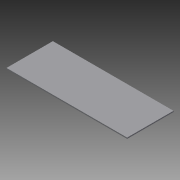
# Autodesk Inventor part: HostPCB
Saved by Autodesk Inventor 2016 (Build 200138000, 138)
## iProperties
Created: 2015-06-09
Part Number: HostPCB
Material: GFRC
Document SubType Name: Modeling
Designer: Yann
Density: 1.7 g/cm^3
Appearance: Flat - Polished Gray
Author: Yann
Autodesk Inventor part; units mm, degrees
ref_plane "YZ Plane" through (0, 0, 0) normal (1, 0, 0) x (0, 1, 0)
ref_plane "XZ Plane" through (0, 0, 0) normal (0, 1, 0) x (-1, 0, 0)
ref_plane "XY Plane" through (0, 0, 0) normal (0, 0, 1) x (1, 0, 0)
sketch "Sketch1" plane through (0, 0, 0) normal (0, 0, 1) x (1, 0, 0)
  line L0 (0, 35) -> (0, -35) construction
  line L1 (-91, 0) -> (91, 0) construction
  line L2 (-65, -25) -> (65, -25)
  line L3 (65, -25) -> (65, 25)
  line L4 (65, 25) -> (-65, 25)
  line L5 (-65, 25) -> (-65, -25)
  line L6 (-65, -25) -> (65, 25) construction
  line L7 (65, -25) -> (-65, 25) construction
  point P0 (0, 0)
  dimension "d0" = 130
  dimension "d1" = 50
  constraints: 12 end point, 2 midpoint, 2 parallel, 1 horizontal, 1 perpendicular
  measures "d0" distance of L4.end L3.end
  measures "d1" distance between parallel lines of L2 L4
extrude "Extrusion1" add sketch "Sketch1" along normal blind 1.2
equation "\"d0\" = HostPCB_Length"
equation "\"d1\" = HostPCB_Width"
equation "\"d2\" = HostPCB_Thickness"
equation "\"Heatsink_Thickness\" = 5"
equation "\"Heatsink_Width\" = 65"
equation "\"Cover_Thickness\" = 2"
equation "\"PowerPCB_Minus_Height\" = 1.2"
equation "\"PowerPCB_Width\" = 63"
equation "\"Interface_Thickness\" = 7"
equation "\"PowerPCB_Thickness\" = 3"
equation "\"PowerPCB_Plus_Height\" = 8"
equation "\"LogicPCB_Width\" = 55"
equation "\"LogicPCB_Thickness\" = 2"
equation "\"LogicPCB_Plus_Height\" = 8"
equation "\"HostPCB_Length\" = 130"
equation "\"HostPCB_Width\" = 50"
equation "\"HostPCB_Plus_Height\" = 8"
equation "\"HostPCB_Thickness\" = 1.2"
body "Solid1"
